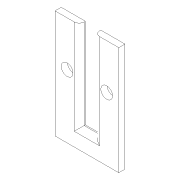
# Autodesk Inventor part: control_arm_hole_guide
Saved by Autodesk Inventor 2022 (Build 260153000, 153)
## iProperties
Created: 2022-08-15
Part Number: control_arm_hole_guide
Material: Generic
Document SubType Name: Modeling
Designer: Thomas
Density: 1 g/cm^3
Appearance: Default
Author: Thomas
Autodesk Inventor part; units mm, degrees
ref_plane "YZ Plane" through (0, 0, 0) normal (1, 0, 0) x (0, 1, 0)
ref_plane "XZ Plane" through (0, 0, 0) normal (0, 1, 0) x (-1, 0, 0)
ref_plane "XY Plane" through (0, 0, 0) normal (0, 0, 1) x (1, 0, 0)
sketch "Sketch1" plane through (0, 0, 0) normal (0, 0, 1) x (1, 0, 0)
  line L0 (0, 0) -> (10.3, 0)
  line L1 (10.3, 0) -> (10.3, 14.5)
  line L2 (10.3, 14.5) -> (0, 14.5)
  line L3 (0, 14.5) -> (0, 0)
  line L4 (3.9, 0) -> (6.4, 0)
  line L5 (6.4, 0) -> (6.4, 14.5)
  line L6 (6.4, 14.5) -> (3.9, 14.5)
  line L7 (3.9, 14.5) -> (3.9, 0)
  line L8 (0, 0) -> (10.3, 0)
  line L9 (10.3, 0) -> (10.3, -3)
  line L10 (10.3, -3) -> (0, -3)
  line L11 (0, -3) -> (0, 0)
  circle A0 centre (1.95, 7.25) radius 0.95
  circle A1 centre (8.35, 7.25) radius 0.95
  dimension "d0" = 10.3
  dimension "d1" = 14.5
  dimension "d2" = 2.5
  dimension "d3" = 3
  dimension "d4" = 3.9
  dimension "d5" = 0
  dimension "d6" = 1.9
  dimension "d7" = 1.95
  dimension "d8" = 7.25
  dimension "d9" = 1.9
  dimension "d10" = 1.95
  dimension "d11" = 7.25
  constraints: 24 end point, 6 parallel, 3 horizontal, 3 perpendicular, 2 centre point, 2 point on line
  measures "d0" distance of L2.end L1.end
  measures "d1" distance of L1.end L0.end
  measures "d2" distance of L6.end L5.end
  measures "d3" distance of L8.end L9.end
  measures "d4" distance between parallel lines of L3 L7
  measures "d5" distance between parallel lines of L2 L6
  measures "d6" diameter of A0
  measures "d7" distance from line of A0.centre L3
  measures "d8" distance from line of L2 A0.centre
  measures "d9" diameter of A1
  measures "d10" distance from line of L1 A1.centre
  measures "d11" distance from line of L2 A1.centre
extrude "Extrusion1" add sketch "Sketch1" along normal blind 1 contours L3 L2 L7 L0 | L0 L9 L10 L11 | L5 L2 L1 L0
fillet "Fillet1" radius 0.8 3 edges at (3.9, 7.25, 1) (5.15, 0, 1) (6.4, 7.25, 1)
equation "\"d4\" = -0.5 * d2 + 0.5 * d0"
equation "\"d7\" = 0.5 * d4"
equation "\"d8\" = 0.5 * d1"
equation "\"d9\" = d6"
equation "\"d10\" = d7"
equation "\"d11\" = d8"
body "Solid1"
